# Autodesk Inventor part: MCP1726
Saved by Autodesk Inventor 2015 SP1 (Build 190203100, 203)
## iProperties
Created: 2015-06-25
Part Number: MCP1726
Material: Generic
Document SubType Name: Modeling
Designer: Patrick
Density: 1 g/cm^3
Appearance: SOIC8, MCP1726
Author: Patrick
Autodesk Inventor part; units mm, degrees
ref_plane "YZ Plane" through (0, 0, 0) normal (1, 0, 0) x (0, 1, 0)
ref_plane "XZ Plane" through (0, 0, 0) normal (0, 1, 0) x (-1, 0, 0)
ref_plane "XY Plane" through (0, 0, 0) normal (0, 0, 1) x (1, 0, 0)
sketch "SOIC8, MCP1726_44" plane through (0, 0, 0) normal (0, 0, 1) x (1, 0, 0)
  line L0 (-3.512, -2.55) -> (-3.512, 2.962)
  line L1 (-3.512, 2.962) -> (3.4, 2.962)
  line L2 (3.4, 2.962) -> (3.4, -2.55)
  line L3 (3.4, -2.55) -> (-3.512, -2.55)
  constraints: 8 end point
extrude "Extrusion1" add sketch "SOIC8, MCP1726_44" along normal blind 1
body "Solid1"
